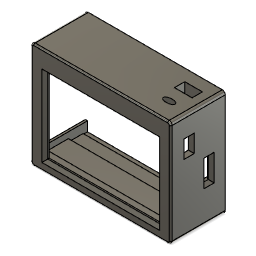
Rasp35inch_housing (Autodesk Fusion 360 design; units mm, degrees)
Autodesk Fusion 360 part; units mm, degrees
sketch "Skizze1" plane through (0, 0, 0) normal (0, 0, 1) x (1, 0, 0)
  line L0 (47.5, 36) -> (-47.5, 36)
  line L1 (-47.5, 36) -> (-47.5, -36)
  line L2 (-47.5, -36) -> (47.5, -36)
  line L3 (47.5, -36) -> (47.5, 36)
  line L4 (47.5, 36) -> (-47.5, -36) construction
  line L5 (-47.5, 36) -> (47.5, -36) construction
  dimension "d1" = 95
  dimension "d2" = 72
  constraint horizontal L0
  constraint perpendicular L0 L1
  constraint parallel L0 L2
  constraint parallel L1 L3
  constraint coincident L4 origin
  constraint coincident L5 origin
  measures "d1" distance of L0.start L0.end
  measures "d2" distance of L0.start L2.end
extrude "Extrusion1" add sketch "Skizze1" along normal blind 40
sketch "Skizze2" plane through (0, 0, 0) normal (0, 0, -1) x (-1, 0, 0)
  line L0 (-47.5, 36) -> (-47.5, -36)
  line L1 (-47.5, -36) -> (47.5, -36)
  line L2 (47.5, -36) -> (47.5, 36)
  line L3 (47.5, 36) -> (-47.5, 36)
  line L4 (38, -29) -> (-38, -29)
  line L5 (-38, -29) -> (-38, 22)
  line L6 (-38, 22) -> (38, 22)
  line L7 (38, 22) -> (38, -29)
  line L8 (38, -29) -> (-38, 22) construction
  line L9 (-38, -29) -> (38, 22) construction
  point P0 (0, -3.5)
  dimension "d5" = 76
  dimension "d6" = 51
  dimension "d8" = 7
  constraint horizontal L4
  constraint perpendicular L4 L5
  constraint parallel L4 L6
  constraint parallel L5 L7
  constraint coincident L8 P0
  constraint coincident L9 P0
  constraint vertical origin P0
  measures "d5" distance of L5.end L6.end
  measures "d6" distance of L4.end L5.end
  measures "d8" distance of L1 L4
extrude "Extrusion2" cut sketch "Skizze2" against normal blind 70 contours L4 L5 L6 L7
sketch "Skizze3" plane through (0, 0, 0) normal (0, 0, -1) x (-1, 0, 0)
  line L0 (-38, -29) -> (-38, 22)
  line L1 (-38, 22) -> (38, 22)
  line L2 (38, 22) -> (38, -29)
  line L3 (38, -29) -> (-38, -29)
  line L4 (-47.5, 36) -> (-47.5, -36)
  line L5 (-47.5, -36) -> (47.5, -36)
  line L6 (47.5, -36) -> (47.5, 36)
  line L7 (47.5, 36) -> (-47.5, 36)
  line L8 (-41.5, 25) -> (44.5, 25)
  line L9 (44.5, 25) -> (44.5, -31)
  line L10 (44.5, -31) -> (-41.5, -31)
  line L11 (-41.5, -31) -> (-41.5, 25)
  line L12 (-41.5, 25) -> (44.5, -31) construction
  line L13 (44.5, 25) -> (-41.5, -31) construction
  point P0 (1.5, -3)
  dimension "d11" = 86
  dimension "d12" = 3
  dimension "d13" = 56
  dimension "d14" = 5
  constraint horizontal L8
  constraint perpendicular L8 L9
  constraint parallel L8 L10
  constraint parallel L9 L11
  constraint coincident L12 P0
  constraint coincident L13 P0
  measures "d11" distance of L8.start L8.end
  measures "d12" distance of L6 L9
  measures "d13" distance of L8.end L9.end
  measures "d14" distance of L5 L10
extrude "Extrusion3" cut sketch "Skizze3" against normal blind 37 contours L8 L9 L10 L11
sketch "Skizze4" plane through (0, 0, 0) normal (0, 0, -1) x (-1, 0, 0)
  line L0 (44.5, 25) -> (44.5, -31)
  line L1 (44.5, -31) -> (-41.5, -31)
  line L2 (-41.5, -31) -> (-41.5, 25)
  line L3 (-41.5, 25) -> (44.5, 25)
  line L4 (-47.5, 36) -> (-47.5, -36)
  line L5 (-47.5, -36) -> (47.5, -36)
  line L6 (47.5, -36) -> (47.5, 36)
  line L7 (47.5, 36) -> (-47.5, 36)
  line L8 (-43.5, 26) -> (46, 26)
  line L9 (46, 26) -> (46, -32)
  line L10 (46, -32) -> (-43.5, -32)
  line L11 (-43.5, -32) -> (-43.5, 26)
  dimension "d18" = 2
  dimension "d19" = 1
  dimension "d20" = 1.5
  dimension "d21" = 1
  constraint horizontal L8
  constraint vertical L9
  constraint horizontal L10
  constraint vertical L11
  measures "d18" distance of L2 L11
  measures "d19" distance of L3 L8
  measures "d20" distance of L0 L9
  measures "d21" distance of L1 L10
extrude "Extrusion4" cut sketch "Skizze4" along normal blind 45 from surface at -31 contours L8 L9 L10 L11
sketch "Skizze5" plane through (0, 0, 0) normal (0, 0, -1) x (-1, 0, 0)
  line L0 (46, -32) -> (-43.5, -32)
  line L1 (-43.5, -32) -> (-43.5, 26)
  line L2 (-43.5, 26) -> (46, 26)
  line L3 (46, 26) -> (46, -32)
  line L4 (-47.5, 36) -> (-47.5, -36)
  line L5 (-47.5, -36) -> (47.5, -36)
  line L6 (47.5, -36) -> (47.5, 36)
  line L7 (47.5, 36) -> (-47.5, 36)
  line L8 (-19, 34.5) -> (-3, 34.5)
  line L9 (-3, 34.5) -> (-3, 25)
  line L10 (-3, 25) -> (-19, 25)
  line L11 (-19, 25) -> (-19, 34.5)
  line L12 (44.5, 25) -> (-41.5, 25)
  line L13 (6, 25) -> (13, 25)
  line L14 (13, 25) -> (13, 28)
  line L15 (13, 28) -> (6, 28)
  line L16 (6, 28) -> (6, 25)
  line L17 (-38, 25) -> (-30, 25)
  line L18 (-30, 25) -> (-30, 28)
  line L19 (-30, 28) -> (-38, 28)
  line L20 (-38, 28) -> (-38, 25)
  dimension "d25" = 22.5
  dimension "d26" = 9.5
  dimension "d27" = 16
  dimension "d31" = 9
  dimension "d32" = 7
  dimension "d33" = 3
  dimension "d34" = 5.5
  dimension "d35" = 8
  dimension "d36" = 3
  constraint horizontal L8
  constraint vertical L9
  constraint horizontal L10
  constraint vertical L11
  constraint collinear L10 L12
  constraint horizontal L13
  constraint vertical L14
  constraint horizontal L15
  constraint vertical L16
  constraint coincident L12 L13.start
  constraint horizontal L17
  constraint vertical L18
  constraint horizontal L19
  constraint vertical L20
  constraint coincident L12 L17.start
  measures "d25" distance of L11 L12.end
  measures "d26" distance of L8.end L9.end
  measures "d27" distance of L8.start L8.end
  measures "d31" distance of L9 L16
  measures "d32" distance of L14.end L15.end
  measures "d33" distance of L13.end L14.end
  measures "d34" distance of L1 L20
  measures "d35" distance of L18.end L19.end
  measures "d36" distance of L17.end L18.end
extrude "Extrusion5" cut sketch "Skizze5" along normal blind 36 from surface at -31 contours L2 L12 L13 L14 L16 | L2 L14 L15 L16 | L2 L18 L19 L20 | L2 L12 L17 L18 L20 | L2 L9 L10 L11 L12 | L2 L8 L9 L11
sketch "Skizze6" plane through (0, 28, 0) normal (0, -1, 0) x (1, 0, 0)
  line L0 (30, 0) -> (38, 0)
  line L1 (38, 0) -> (38, 31)
  line L2 (38, 31) -> (30, 31)
  line L3 (30, 31) -> (30, 0)
  ellipse E0 centre (34, 27.5) end of major axis (38, 27.5) minor radius 2
  line L4 (30, 27.5) -> (38, 27.5)
  line L5 (34, 25.5) -> (34, 29.5)
  line L6 (40, 18) -> (28, 18)
  line L7 (28, 18) -> (28, 11)
  line L8 (28, 11) -> (40, 11)
  line L9 (40, 11) -> (40, 18)
  line L10 (40, 18) -> (28, 11) construction
  line L11 (28, 18) -> (40, 11) construction
  point P0 (34, 14.5)
  dimension "d37" = 4
  dimension "d38" = 1.5
  dimension "d46" = 12
  dimension "d47" = 7
  dimension "d48" = 13
  constraint parallel L2 L4
  constraint coincident E0 L4.start
  constraint coincident E0 L4.end
  constraint coincident E0 L5.start
  constraint coincident E0 L5.end
  constraint coincident L1 L4.end
  constraint coincident L3 L4.start
  constraint horizontal L6
  constraint perpendicular L6 L7
  constraint parallel L6 L8
  constraint parallel L7 L9
  constraint coincident L10 P0
  constraint coincident L11 P0
  constraint vertical E0.centre P0
  measures "d37" distance of E0
  measures "d38" distance of L2 L5.end
  measures "d46" distance of L6.start L6.end
  measures "d47" distance of L6.start L8.end
  measures "d48" distance of E0.centre P0
extrude "Extrusion6" cut sketch "Skizze6" along normal blind -11 and the other way blind -8 contours L3 L6 L7 L8 | L1 L3 L6 L8 | L1 L6 L8 L9 | E0 L4 L5 | E0 L4 L5 | E0 L4 L5 | E0 L4 L5
sketch "Skizze7" plane through (43.5, 0, 0) normal (-1, 0, 0) x (0, 0, 1)
  line L0 (0, 26) -> (0, -32)
  line L1 (0, -32) -> (31, -32)
  line L2 (31, -32) -> (31, 26)
  line L3 (31, 26) -> (0, 26)
  line L4 (31, 22) -> (24, 22)
  line L5 (24, 22) -> (24, 10)
  line L6 (24, 10) -> (31, 10)
  line L7 (31, 10) -> (31, 22)
  dimension "d41" = 4
  dimension "d42" = 12
  dimension "d43" = 7
  constraint horizontal L4
  constraint vertical L5
  constraint horizontal L6
  constraint vertical L7
  constraint coincident L2 L4.start
  measures "d41" distance of L3 L4
  measures "d42" distance of L4.end L5.end
  measures "d43" distance of L5.end L6.end
extrude "Extrusion7" cut sketch "Skizze7" against normal blind 8 contours L2 L4 L5 L6 L7
sketch "Skizze8" plane through (0, 0, 0) normal (0, 0, -1) x (-1, 0, 0)
  line L0 (-3, 34.5) -> (-3, 26)
  line L1 (-3, 26) -> (6, 26)
  line L2 (6, 26) -> (6, 28)
  line L3 (6, 28) -> (13, 28)
  line L4 (13, 28) -> (13, 26)
  line L5 (13, 26) -> (46, 26)
  line L6 (46, 26) -> (46, -32)
  line L7 (46, -32) -> (-43.5, -32)
  line L8 (-43.5, -32) -> (-43.5, 26)
  line L9 (-43.5, 26) -> (-38, 26)
  line L10 (-38, 26) -> (-38, 28)
  line L11 (-38, 28) -> (-30, 28)
  line L12 (-30, 28) -> (-30, 26)
  line L13 (-30, 26) -> (-19, 26)
  line L14 (-19, 26) -> (-19, 34.5)
  line L15 (-19, 34.5) -> (-3, 34.5)
  line L16 (-47.5, 36) -> (-47.5, -36)
  line L17 (-47.5, -36) -> (47.5, -36)
  line L18 (47.5, -36) -> (47.5, 36)
  line L19 (47.5, 36) -> (-47.5, 36)
  line L20 (-43.5, 26) -> (46, 26)
  line L21 (46, 26) -> (46, -34)
  line L22 (46, -34) -> (-43.5, -34)
  line L23 (-43.5, -34) -> (-43.5, 26)
  dimension "d51" = 2
  constraint horizontal L20
  constraint vertical L21
  constraint horizontal L22
  constraint vertical L23
  constraint collinear L5 L20
  constraint collinear L8 L23
  constraint collinear L6 L21
  measures "d51" distance of L7 L22
extrude "Extrusion8" cut sketch "Skizze8" along normal blind 35 from surface at -16 contours L7 L21 L22 L23
sketch "Skizze9" plane through (-46, 0, 0) normal (1, 0, 0) x (0, 0, -1)
  line L0 (0, -34) -> (0, 26)
  line L1 (0, 26) -> (-31, 26)
  line L2 (-31, 26) -> (-31, -32)
  line L3 (-31, -32) -> (-16, -32)
  line L4 (-16, -32) -> (-16, -34)
  line L5 (-16, -34) -> (0, -34)
  line L6 (-31, 25) -> (0, 25)
  line L7 (0, 25) -> (0, -28)
  line L8 (0, -28) -> (-31, -28)
  line L9 (-31, -28) -> (-31, 25)
  line L10 (-31, 25) -> (-37, 25)
  dimension "d56" = 53
  constraint horizontal L6
  constraint vertical L7
  constraint horizontal L8
  constraint vertical L9
  constraint coincident L0 L7.end
  constraint coincident L2 L6.start
  constraint coincident L6.start L9.end
  measures "d56" distance of L6.end L7.end
extrude "Extrusion9" cut sketch "Skizze9" against normal blind 3 contours L0 L2 L6 L7 L8 L9
sketch "Skizze10" plane through (0, 0, 0) normal (0, 0, -1) x (-1, 0, 0)
  line L0 (46, 25) -> (47.5, 25)
  line L1 (47.5, 25) -> (47.5, 36)
  line L2 (47.5, 36) -> (-47.5, 36)
  line L3 (-47.5, 36) -> (-47.5, -36)
  line L4 (-47.5, -36) -> (47.5, -36)
  line L5 (47.5, -36) -> (47.5, -28)
  line L6 (47.5, -28) -> (46, -28)
  line L7 (46, -28) -> (46, -34)
  line L8 (46, -34) -> (-43.5, -34)
  line L9 (-43.5, -34) -> (-43.5, 26)
  line L10 (-43.5, 26) -> (-38, 26)
  line L11 (-38, 26) -> (-38, 28)
  line L12 (-38, 28) -> (-30, 28)
  line L13 (-30, 28) -> (-30, 26)
  line L14 (-30, 26) -> (-19, 26)
  line L15 (-19, 26) -> (-19, 34.5)
  line L16 (-19, 34.5) -> (-3, 34.5)
  line L17 (-3, 34.5) -> (-3, 26)
  line L18 (-3, 26) -> (6, 26)
  line L19 (6, 26) -> (6, 28)
  line L20 (6, 28) -> (13, 28)
  line L21 (13, 28) -> (13, 26)
  line L22 (13, 26) -> (46, 26)
  line L23 (46, 26) -> (46, 25)
  line L24 (-46, 34.5) -> (46, 34.5)
  line L25 (46, 34.5) -> (46, -34.5)
  line L26 (-46, -34.5) -> (-46, 34.5)
  line L27 (-46, -34.5) -> (46, -34.5)
  dimension "d59" = 1.5
  dimension "d60" = 1.5
  dimension "d61" = 1.5
  constraint horizontal L24
  constraint vertical L25
  constraint vertical L26
  constraint perpendicular L25 L27
  measures "d59" distance of L2 L24
  measures "d60" distance of L3 L26
  measures "d61" distance of L4 L27
extrude "Extrusion10" cut sketch "Skizze10" against normal blind 6 contours L17 L18 L19 L20 L21 L22 L24 L25 | L8 L9 L10 L11 L12 L13 L14 L15 L24 L25 L26 L27
extrude "Extrusion11" cut 1 faces at (15.3333, -35.5, 0) along direction (0, 0, 1) blind 3
fillet "Abrundung1" radius 2 4 edges at (-47.5, -36, 21.5) (-47.5, 36, 21.5) (47.5, 36, 21.5) (47.5, -36, 21.5)
chamfer "Fase1" distance 2 angle 45 4 edges at (0, 22, 40) (-38, -3.5, 40) (38, -3.5, 40) (0, -29, 40)
fillet "Abrundung2" radius 1 8 edges at (46.9142, -35.4142, 40) (47.5, 0, 40) (46.9142, 35.4142, 40) (0, 36, 40) (-46.9142, 35.4142, 40) (-47.5, 0, 40) (-46.9142, -35.4142, 40) (0, -36, 40)
sketch "Skizze11" plane through (43.5, 0, 0) normal (-1, 0, 0) x (0, 0, 1)
  line L0 (6, 26) -> (6, -34)
  line L1 (6, -34) -> (16, -34)
  line L2 (16, -34) -> (16, -32)
  line L3 (16, -32) -> (31, -32)
  line L4 (31, -32) -> (31, 10)
  line L5 (31, 10) -> (24, 10)
  line L6 (24, 10) -> (24, 22)
  line L7 (24, 22) -> (31, 22)
  line L8 (31, 22) -> (31, 26)
  line L9 (31, 26) -> (6, 26)
  line L10 (12.5, 2) -> (15.5, 2)
  line L11 (15.5, 2) -> (15.5, -12)
  line L12 (15.5, -12) -> (12.5, -12)
  line L13 (12.5, -12) -> (12.5, 2)
  dimension "d71" = 0.5
  dimension "d72" = 14
  dimension "d73" = 22
  dimension "d74" = 3
  constraint horizontal L10
  constraint vertical L11
  constraint horizontal L12
  constraint vertical L13
  measures "d71" distance of L2 L11
  measures "d72" distance of L10.start L12.end
  measures "d73" distance of L1 L12
  measures "d74" distance of L10.start L10.end
extrude "Extrusion12" cut sketch "Skizze11" against normal blind 8 contours L10 L11 L12 L13
chamfer "Fase2" distance 2 angle 45 4 edges at (47.5, -5, 15.5) (47.5, -5, 12.5) (47.5, -12, 14) (47.5, 2, 14)
sketch "Skizze12" plane through (0, 0, 6) normal (0, 0, -1) x (-1, 0, 0)
  line L0 (-46, 34.5) -> (-46, -34.5)
  line L1 (-46, -34.5) -> (46, -34.5)
  line L2 (46, -34.5) -> (46, -34)
  line L3 (46, -34) -> (-43.5, -34)
  line L4 (-43.5, -34) -> (-43.5, 26)
  line L5 (-43.5, 26) -> (-38, 26)
  line L6 (-38, 26) -> (-38, 28)
  line L7 (-38, 28) -> (-30, 28)
  line L8 (-30, 28) -> (-30, 26)
  line L9 (-30, 26) -> (-19, 26)
  line L10 (-19, 26) -> (-19, 34.5)
  line L11 (-19, 34.5) -> (-46, 34.5)
  line L12 (-43.5, 2) -> (-45, 2)
  line L13 (-45, 2) -> (-45, -12)
  line L14 (-45, -12) -> (-43.5, -12)
  line L15 (-43.5, -12) -> (-43.5, 2)
  line L16 (-43.5, 2) -> (-43.5, -12)
  dimension "d78" = 1.5
  constraint horizontal L12
  constraint vertical L13
  constraint horizontal L14
  constraint vertical L15
  constraint coincident L4 L12.start
  constraint coincident L12.start L15.end
  constraint coincident L14.end L15.start
  measures "d78" distance of L12.start L12.end
extrude "Extrusion13" cut sketch "Skizze12" against normal blind 9 contours L4 L12 L13 L14 L15 L16
equation "d16 = -40.00 mm + 3 mm"
equation "d60 = d59"
